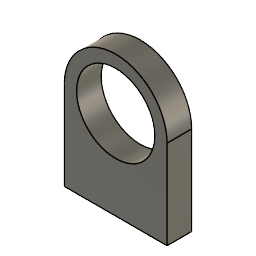
Radial Bearing Stand (Autodesk Fusion 360 design; units mm, degrees)
part number: 2026-05-13-22-26-53-458
Autodesk Fusion 360 part; units mm, degrees
sketch "Sketch1" plane through (0, 0, 0) normal (0, 0, 1) x (1, 0, 0)
  line L0 (12.5, -3) -> (-12.5, -3)
  line L1 (-12.5, -3) -> (-12.5, 3)
  line L2 (-12.5, 3) -> (12.5, 3)
  line L3 (12.5, 3) -> (12.5, -3)
  line L4 (12.5, -3) -> (-12.5, 3) construction
  line L5 (-12.5, -3) -> (12.5, 3) construction
  dimension "d1" = 6
  dimension "d2" = 25
  constraint horizontal L0
  constraint perpendicular L0 L1
  constraint parallel L0 L2
  constraint parallel L1 L3
  constraint coincident L4 origin
  constraint coincident L5 origin
  measures "d1" distance of L0.end L1.end
  measures "d2" distance of L0.start L0.end
extrude "Extrude1" add sketch "Sketch1" along normal blind 21.616
sketch "Sketch2" plane through (0, -3, 0) normal (0, -1, 0) x (1, 0, 0)
  line L0 (-12.5, 0) -> (12.5, 0)
  line L1 (12.5, 0) -> (12.5, 21.616)
  line L2 (12.5, 21.616) -> (-12.5, 21.616)
  line L3 (-12.5, 21.616) -> (-12.5, 0)
  circle A0 centre (0, 21.616) radius 12.5
  circle A1 centre (0, 21.616) radius 9.5
  dimension "d5" = 19
  constraint midpoint L2 A0.centre
  constraint coincident L1.end A0
  constraint concentric A0 A1
  measures "d5" diameter of A1
extrude "Extrude2" add sketch "Sketch2" against normal blind 6 contours L2 A0 A1 picked at (-11.4535, 22.237)
extrude "Extrude3" cut sketch "Sketch2" against normal blind 6 contours L2 A1 picked at (0.2366, 18.4582)
